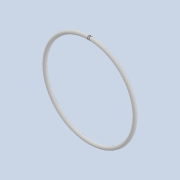
# Autodesk Inventor part: Wire
Saved by Autodesk Inventor 2020.4 (Build 244396000, 396)
## iProperties
Created: 2020-05-04
Part Number: Wire
Material: Generic
Document SubType Name: Modeling
Designer: Acer
Density: 1 g/cm^3
Appearance: Default
Author: Acer
Autodesk Inventor part; units mm, degrees
ref_plane "YZ Plane" through (0, 0, 0) normal (1, 0, 0) x (0, 1, 0)
ref_plane "XZ Plane" through (0, 0, 0) normal (0, 1, 0) x (-1, 0, 0)
ref_plane "XY Plane" through (0, 0, 0) normal (0, 0, 1) x (1, 0, 0)
sketch "Sketch1" plane through (0, 0, 0) normal (0, 0, 1) x (1, 0, 0)
  circle A0 centre (0, 0) radius 20.4
  dimension "d0" = 40.8
  constraints: 1 centre point, 1 coincident
  measures "d0" diameter of A0
sketch "Sketch2" plane through (0, 0, 0) normal (0, 1, 0) x (-1, 0, 0)
  line L0 (20.4, 0) -> (-20.4, 0) projected
  circle A0 centre (20.4, 0) radius 0.825
  point P0 (0, 0)
  dimension "d1" = 1.65
  constraints: 1 centre point, 1 coincident
  measures "d1" diameter of A0
sweep "Sweep1" add profiles "Sketch2" path "Sketch1"
sketch "Sketch3" plane through (0, 0, 0) normal (1, 0, 0) x (0, 1, 0)
  arc A0 (20.4, -0.825) -> (20.4, 0.825) centre (20.4, 0) ccw projected
  arc A1 (20.4, 0.825) -> (20.4, -0.825) centre (20.4, 0) ccw projected
  circle A2 centre (20.4, 0) radius 1
  point P0 (0, 0)
  dimension "d4" = 2
  constraints: 1 centre point, 1 coincident
  measures "d4" diameter of A2
extrude "Extrusion1" cut sketch "Sketch3" along normal mid plane 0.75 contours A1 A0 | A2
body "Solid1"
